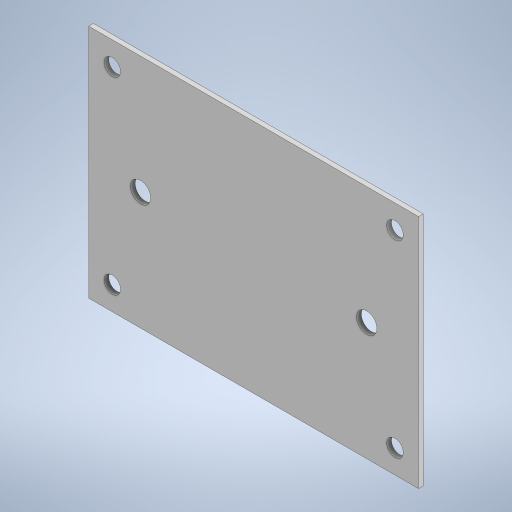
# Autodesk Inventor part: DCDCconvertor_plate
Saved by Autodesk Inventor 2023 (Build 270158000, 158)
## iProperties
Created: 2023-10-03
Part Number: DCDCconvertor_plate
Material: Generic
Document SubType Name: Sheet Metal
Designer: 310611102
Density: 1 g/cm^3
Sheet Metal Rule: Default_mm
Appearance: Default
Author: 310611102
Autodesk Inventor part; units mm, degrees
ref_plane "YZ Plane" through (0, 0, 0) normal (1, 0, 0) x (0, 1, 0)
ref_plane "XZ Plane" through (0, 0, 0) normal (0, 1, 0) x (-1, 0, 0)
ref_plane "XY Plane" through (0, 0, 0) normal (0, 0, 1) x (1, 0, 0)
sketch "Sketch1" plane through (0, 0, 0) normal (0, 0, 1) x (1, 0, 0)
  line L0 (-35, 25) -> (35, 25)
  line L1 (35, 25) -> (35, -25)
  line L2 (35, -25) -> (-35, -25)
  line L3 (-35, -25) -> (-35, 25)
  line L4 (-35, 25) -> (35, -25) construction
  line L5 (35, 25) -> (-35, -25) construction
  circle A0 centre (-24, 0) radius 2.15
  circle A1 centre (24, 0) radius 2.15
  circle A2 centre (-30, 20) radius 1.75
  line L6 (0, 13.5327) -> (0, 0) construction
  line L7 (0, 0) -> (11.3828, 0) construction
  circle A3 centre (30, 20) radius 1.75
  circle A4 centre (-30, -20) radius 1.75
  circle A5 centre (30, -20) radius 1.75
  dimension "d0" = 50
  dimension "d1" = 70
  dimension "d2" = 48
  dimension "d3" = 24
  dimension "d4" = 4.3
  dimension "d6" = 3.5
  dimension "d10" = 5
  dimension "d11" = 5
  constraints: 16 end point, 6 centre point, 3 symmetric about line, 2 horizontal, 2 horizontal alignment, 2 midpoint, 2 parallel, 1 equal radius, 1 perpendicular, 1 vertical, 3 other
  measures "d0" distance of L0.end L1.end
  measures "d1" distance of L0.start L0.end
  measures "d2" distance of A1.centre A0.centre
  measures "d3" distance of L6.end A0.centre
  measures "d4" diameter of A0
  measures "d6" diameter of A2
  measures "d10" distance from line of L3 A2.centre
  measures "d11" distance from line of L0 A2.centre
extrude "Plate1" add sketch "Sketch1" along normal blind 1
equation "\"d3\" = 0.5 * d2"
equation "\"d5\" = 厚度"
equation "\"折彎半徑\" = 厚度"
equation "\"折彎離隙寬度\" = 厚度"
equation "\"折彎離隙深度\" = 0.5 * 厚度"
equation "\"轉角離隙大小\" = 4 * 厚度"
equation "\"最小剩餘\" = 2 * 厚度"
equation "\"轉移半徑\" = 折彎半徑"
equation "\"Jacobi半徑大小\" = 折彎半徑"
equation "\"間隙大小\" = 厚度"
equation "\"厚度\" = 1"
body "Solid1"
